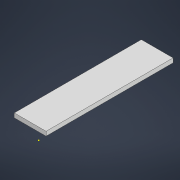
# Autodesk Inventor part: sensorbar
Saved by Autodesk Inventor 2022 (Build 260153000, 153)
## iProperties
Created: 2021-10-11
Part Number: sensorbar
Material: 一般
Document SubType Name: Modeling
Designer: shiok
Density: 1 g/cm^3
Appearance: 既定
Author: shiok
Autodesk Inventor part; units mm, degrees
ref_plane "YZ Plane" through (0, 0, 0) normal (1, 0, 0) x (0, 1, 0)
ref_plane "XZ Plane" through (0, 0, 0) normal (0, 1, 0) x (-1, 0, 0)
ref_plane "XY Plane" through (0, 0, 0) normal (0, 0, 1) x (1, 0, 0)
sketch "スケッチ1" plane through (0, 0, 0) normal (0, 1, 0) x (-1, 0, 0)
  line L0 (-4.0796, -3.4942) -> (-19.0796, -3.4942)
  line L1 (-19.0796, -3.4942) -> (-19.0796, -63.4942)
  line L2 (-19.0796, -63.4942) -> (-4.0796, -63.4942)
  line L3 (-4.0796, -63.4942) -> (-4.0796, -3.4942)
  dimension "d0" = 15
  dimension "d1" = 60
  constraints: 8 end point, 2 parallel, 1 horizontal, 1 perpendicular
  measures "d0" distance of L2.end L1.end
  measures "d1" distance of L1.end L0.end
extrude "押し出し1" add sketch "スケッチ1" along normal blind 2
sketch "スケッチ2" plane through (19.0796, 0, -3.4942) normal (1, 0, 0) x (0, 0, -1)
  point P0 (-3.4942, 0)
